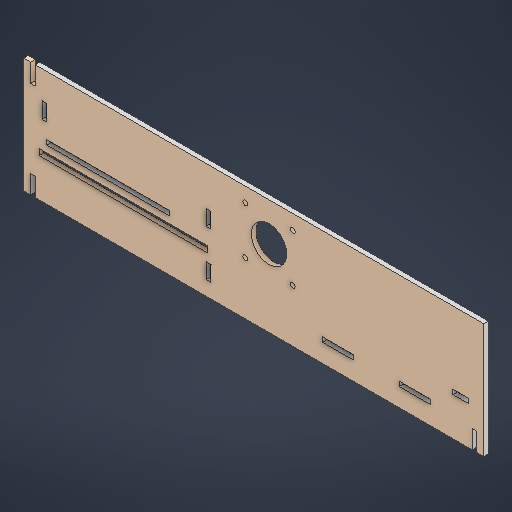
# Autodesk Inventor part: Sideboard
Saved by Autodesk Inventor 2027 (Build 310192000, 192)
## iProperties
Created: 2026-05-09
Part Number: Sideboard
Material: Generic
Document SubType Name: Modeling
Designer: alexy
Density: 1 g/cm^3
Appearance: Default
Author: alexy
Autodesk Inventor part; units mm, degrees
ref_plane "YZ Plane" through (0, 0, 0) normal (1, 0, 0) x (0, 1, 0)
ref_plane "XZ Plane" through (0, 0, 0) normal (0, 1, 0) x (-1, 0, 0)
ref_plane "XY Plane" through (0, 0, 0) normal (0, 0, 1) x (1, 0, 0)
sketch "Sketch1" plane through (0, 0, 0) normal (0, 0, 1) x (1, 0, 0)
  line L0 (0, 0) -> (300, 0)
  line L1 (300, 0) -> (300, 65)
  line L2 (300, 65) -> (0, 65)
  line L3 (0, 65) -> (0, 0)
  circle A0 centre (144.5, 55.5) radius 1.55
  circle A1 centre (144.5, 24.5) radius 1.55
  circle A2 centre (175.5, 55.5) radius 1.55
  circle A3 centre (175.5, 24.5) radius 1.55
  circle A4 centre (160, 40) radius 11.5
  line L4 (10, 19) -> (120, 19)
  line L5 (120, 19) -> (120, 15)
  line L6 (120, 15) -> (10, 15)
  line L7 (10, 15) -> (10, 19)
  line L8 (0, 65) -> (39.6145, 65)
  line L9 (7.5, 53) -> (4.5, 53)
  line L10 (4.5, 53) -> (4.5, 65)
  line L11 (4.5, 65) -> (7.5, 65)
  line L12 (7.5, 65) -> (7.5, 53)
  line L13 (7.5, 53) -> (4.5, 65) construction
  line L14 (4.5, 53) -> (7.5, 65) construction
  line L15 (0, 65) -> (50, 65)
  line L16 (0, 0) -> (0, -10)
  line L17 (0, -10) -> (300, -10)
  line L18 (300, -10) -> (300, 0)
  point P0 (6, 59)
  point P1 (4.5, 59)
  point P2 (7.5, 59)
  point P3 (10, 17)
  point P4 (120, 17)
  dimension "d1" = 3.1
  dimension "d2" = 3.1
  dimension "d3" = 3.1
  dimension "d4" = 3.1
  dimension "d5" = 31
  dimension "d7" = 23
  dimension "d8" = 15.5
  dimension "d9" = 15.5
  dimension "d10" = 65
  dimension "d11" = 31
  dimension "d13" = 40
  dimension "d54" = 300
  dimension "d55" = 3
  dimension "d56" = 4.5
  dimension "d59" = 110
  dimension "d93" = 15
  dimension "d107" = 10
  dimension "d201" = 4
  dimension "d202" = 10
  dimension "d274" = 12
  dimension "d287" = 140
  constraints: 38 end point, 6 midpoint, 6 parallel, 5 centre point, 5 perpendicular, 4 horizontal, 3 horizontal alignment, 2 vertical alignment, 1 vertical
  measures "d1" diameter of A0
  measures "d2" diameter of A1
  measures "d3" diameter of A2
  measures "d4" diameter of A3
  measures "d5" distance of A1.centre A3.centre
  measures "d7" diameter of A4
  measures "d8" horizontal distance of A0.centre A4.centre
  measures "d9" horizontal distance of A4.centre A3.centre
  measures "d10" distance of L0.end L1.end
  measures "d11" distance of A3.centre A2.centre
  measures "d13" distance from line of L0 A4.centre
  measures "d54" distance of L0.end L0.start
  measures "d55" distance of L10.end L11.end
  measures "d56" distance between parallel lines of L3 L10
  measures "d59" distance of L5.end L6.end
  measures "d93" distance between parallel lines of L0 L6
  measures "d107" distance from line of L3 point (10, 17)
  measures "d201" distance of L6.end L4.start
  measures "d202" distance of L0.start L16.end
  measures "d274" distance from line of L15 L9.start
  measures "d287" distance from line of L1 A4.centre
extrude "Extrusion1" add sketch "Sketch1" along normal blind 3 contours L3 L2 L10 L9 L12 L1 L0 | L0 L18 L17 L16
sketch "Sketch7" plane through (0, 0, 3) normal (0, 0, 1) x (1, 0, 0)
  line L0 (300, 65) -> (0, 65) projected
  circle A0 centre (144.5, 55.5) radius 1.55 projected
  line L1 (118.95, 39.55) -> (122.05, 39.55)
  line L2 (122.05, 39.55) -> (122.05, 29.45)
  line L3 (122.05, 29.45) -> (118.95, 29.45)
  line L4 (118.95, 29.45) -> (118.95, 39.55)
  line L5 (118.95, 39.55) -> (122.05, 29.45) construction
  line L6 (122.05, 39.55) -> (118.95, 29.45) construction
  line L7 (122.1, 9.55) -> (122.1, -0.55)
  line L8 (122.1, -0.55) -> (118.9, -0.55)
  line L9 (118.9, 9.55) -> (122.1, 9.55)
  line L10 (118.9, -0.55) -> (118.9, 9.55)
  line L11 (118.9, 9.55) -> (122.1, -0.55) construction
  line L12 (122.1, 9.55) -> (118.9, -0.55) construction
  line L13 (0, -10) -> (300, -10) projected
  line L14 (300, -10) -> (300, 65) projected
  circle A1 centre (144.5, 24.5) radius 1.55 projected
  point P0 (0, 0)
  point P1 (242, 62)
  point P2 (120.5, 34.5)
  point P3 (120.5, 4.5)
  point P4 (118.9, 4.5)
  point P5 (150, -10)
  dimension "d185" = 3.2
  dimension "d271" = 3.1
  dimension "d273" = 30
  dimension "d275" = 24
  constraints: 24 end point, 6 midpoint, 4 parallel, 2 horizontal, 2 perpendicular, 1 other
  measures "d185" distance of L7.end L12.end
  measures "d271" distance of L1.start L1.end
  measures "d273" distance of point (120.5, 4.5) point (120.5, 34.5)
  measures "d275" horizontal distance of A1.centre point (120.5, 34.5)
extrude "Extrusion6" cut sketch "Sketch7" against normal blind 3 contours L1 L2 L3 L4 | L7 L8 L10 L9
sketch "Sketch8" plane through (0, 0, 3) normal (0, 0, 1) x (1, 0, 0)
  line L0 (0, -10) -> (300, -10) projected
  line L1 (279.95, 18) -> (290, 18)
  line L2 (290, 18) -> (290, 14.95)
  line L3 (290, 14.95) -> (279.95, 14.95)
  line L4 (279.95, 14.95) -> (279.95, 18)
  line L5 (300, -10) -> (300, 65) projected
  line L6 (4.5, 2) -> (7.5, 2)
  line L7 (7.5, 2) -> (7.5, -10)
  line L8 (7.5, -10) -> (4.5, -10)
  line L9 (4.5, -10) -> (4.5, 2)
  line L10 (4.5, 2) -> (7.5, -10) construction
  line L11 (7.5, 2) -> (4.5, -10) construction
  line L12 (295.5, 2) -> (292.5, 2)
  line L13 (292.5, 2) -> (292.5, -10)
  line L14 (292.5, -10) -> (295.5, -10)
  line L15 (295.5, -10) -> (295.5, 2)
  line L16 (295.5, 2) -> (292.5, -10) construction
  line L17 (292.5, 2) -> (295.5, -10) construction
  point P0 (0, 0)
  point P1 (6, -4)
  point P2 (4.5, -4)
  point P3 (294, -4)
  dimension "d219" = 28
  dimension "d220" = 3.05
  dimension "d221" = 10.05
  dimension "d222" = 10
  dimension "d223" = 3
  dimension "d247" = 3
  dimension "d248" = 6
  dimension "d249" = 12
  dimension "d263" = 6
  constraints: 32 end point, 6 parallel, 5 midpoint, 3 horizontal, 3 perpendicular, 2 horizontal alignment, 1 point on line
  measures "d219" distance between parallel lines of L0 L1
  measures "d220" distance of L3.end L1.start
  measures "d221" distance of L2.end L3.end
  measures "d222" distance between parallel lines of L5 L2
  measures "d223" distance of L7.end L8.end
  measures "d247" distance between parallel lines of L13 L15
  measures "d248" distance from line of L5 point (294, -4)
  measures "d249" distance of L14.end L12.start
  measures "d263" horizontal distance of L0.start point (6, -4)
extrude "Extrusion7" cut sketch "Sketch8" against normal blind 3
sketch "Sketch11" plane through (0, 0, 0) normal (0, 0, -1) x (-1, 0, 0)
  line L0 (-12, 47) -> (-15.05, 47)
  line L1 (-15.05, 47) -> (-15.05, 36.5)
  line L2 (-15.05, 36.5) -> (-12, 36.5)
  line L3 (-12, 36.5) -> (-12, 47)
  line L4 (0, 65) -> (0, -10) projected
  line L5 (-300, 65) -> (-7.5, 65) projected
  line L6 (-95.15, 26.5) -> (-15.05, 26.5)
  line L7 (-15.05, 26.5) -> (-15.05, 23.45)
  line L8 (-15.05, 23.45) -> (-95.15, 23.45)
  line L9 (-95.15, 23.45) -> (-95.15, 26.5)
  point P0 (0, 0)
  point P1 (-12, 41.75)
  dimension "d276" = 12
  dimension "d277" = 18
  dimension "d278" = 10.5
  dimension "d279" = 3.05
  dimension "d282" = 10
  dimension "d283" = 80.1
  dimension "d284" = 3.05
  constraints: 16 end point, 4 parallel, 2 horizontal, 2 perpendicular, 1 midpoint, 1 vertical alignment
  measures "d276" distance from line of L4 point (-12, 41.75)
  measures "d277" distance from line of L5 L0.start
  measures "d278" distance of L2.end L0.start
  measures "d279" distance of L0.start L0.end
  measures "d282" distance of L6.end L1.end
  measures "d283" distance of L7.end L8.end
  measures "d284" distance of L6.end L7.end
extrude "Extrusion9" cut sketch "Sketch11" against normal blind 3
sketch "Sketch12" plane through (0, 0, 3) normal (0, 0, 1) x (1, 0, 0)
  line L0 (194.85, 5.05) -> (214.95, 5.05)
  line L1 (214.95, 5.05) -> (214.95, 2)
  line L2 (214.95, 2) -> (194.85, 2)
  line L3 (194.85, 2) -> (194.85, 5.05)
  line L4 (244.95, 5.05) -> (265, 5.05)
  line L5 (265, 5.05) -> (265, 2)
  line L6 (265, 2) -> (244.95, 2)
  line L7 (244.95, 2) -> (244.95, 5.05)
  point P0 (0, 0)
  point P1 (300, -10)
  dimension "d288" = 3.05
  dimension "d289" = 20.05
  dimension "d290" = 20.1
  dimension "d291" = 30
  dimension "d292" = 35
  dimension "d293" = 12
  constraints: 16 end point, 4 parallel, 2 horizontal, 2 horizontal alignment, 2 perpendicular
  measures "d288" distance of L4.end L5.end
  measures "d289" distance of L5.end L6.end
  measures "d290" distance of L1.end L2.end
  measures "d291" distance of L6.end L1.end
  measures "d292" horizontal distance of point (300, -10) L5.end
  measures "d293" vertical distance of point (300, -10) L5.end
extrude "Extrusion10" cut sketch "Sketch12" against normal blind 3
body "Solid1"
